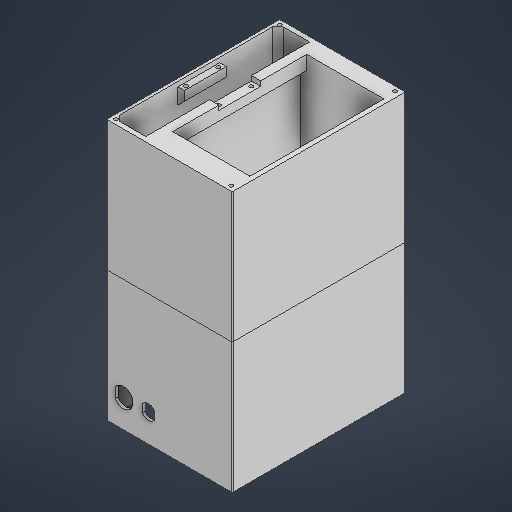
# Autodesk Inventor part: Kameraturm
Saved by Autodesk Inventor 2026.1 (Build 301233020, 233B)
## iProperties
Created: 2025-08-17
Part Number: Kameraturm
Material: Generic
Document SubType Name: Modeling
Designer: peter
Density: 1 g/cm^3
Appearance: Default
Author: peter
Autodesk Inventor part; units mm, degrees
ref_plane "YZ Plane" through (0, 0, 0) normal (1, 0, 0) x (0, 1, 0)
ref_plane "XZ Plane" through (0, 0, 0) normal (0, 1, 0) x (-1, 0, 0)
sketch "Sketch1" plane through (0, 0, 0) normal (0, 0, 1) x (1, 0, 0)
  line L0 (-67.5, -90) -> (67.5, -90)
  line L1 (67.5, -90) -> (67.5, 93)
  line L2 (67.5, 93) -> (-67.5, 93)
  line L3 (-67.5, 93) -> (-67.5, -90)
  line L4 (67.5, -90) -> (-67.5, -90)
  line L5 (-67.5, -90) -> (-67.5, -93)
  line L6 (-67.5, -93) -> (67.5, -93)
  line L7 (67.5, -93) -> (67.5, -90)
  line L8 (-67, -93) -> (-67.5, -92.5) projected
  line L9 (-67, -93) -> (67, -93) projected
  line L10 (67.5, -92.5) -> (67, -93) projected
  line L11 (67.5, -92.5) -> (67.5, 92.5) projected
  line L12 (67, 93) -> (67.5, 92.5) projected
  line L13 (67, 93) -> (-67, 93) projected
  line L14 (-67.5, 92.5) -> (-67, 93) projected
  line L15 (-67.5, 92.5) -> (-67.5, -92.5) projected
  circle A0 centre (57.5, 84) radius 7.05 projected
  circle A1 centre (57.5, -84) radius 7.05 projected
  circle A2 centre (-47.5, 0) radius 7.05 projected
  line L16 (62.5, 75) -> (62.5, -69) projected
  line L17 (62.5, -69) -> (-27.5, -69) projected
  line L18 (-27.5, -69) -> (-27.5, 75) projected
  line L19 (-27.5, 75) -> (62.5, 75) projected
  point P0 (0, 0)
  dimension "d17" = 3
  constraints: 16 end point, 4 parallel, 2 horizontal, 2 perpendicular, 1 coincident
  measures "d17" distance of L5.end L4.end
extrude "Extrusion1" add sketch "Sketch1" along normal blind 280 contours L3 L14 L2 L12 L1 L0 A1 | L0 A1 L7 L10 L6 L8 L5 | A1 L0 | L0 A1 | L3 L2 L14 | L8 L6 L5 | L2 L1 L12 | L10 L7 L6 | A0 | A2 | L16 L17 L18 L19
sketch "Sketch2" plane through (-67.5, -93, 0) normal (0, -1, 0) x (1, 0, 0)
  circle A0 centre (18, -18) radius 10.35 projected
  circle A1 centre (45, -18) radius 7.85 projected
  line L0 (18, -18) -> (18, 64.5706) construction
  line L1 (45, -18) -> (45, 64.5706) construction
  line L2 (40, 0) -> (40, 300) construction
  circle A2 centre (18, 30) radius 10.35
  circle A3 centre (45, 30) radius 7.85
  line L3 (0, 0) -> (135, 0) construction
  point P0 (67.5, 0)
  dimension "d2" = 30
  constraints: 4 end point, 2 centre point, 2 equal radius, 2 point on line, 1 horizontal alignment, 1 parallel, 1 vertical
  measures "d2" distance from line of L3 A2.centre
extrude "Extrusion3" cut sketch "Sketch2" against normal blind 8 contours A2 | A3
ref_plane "Work Plane2" through (0, 0, 34) normal (0, 0, -1) x (-1, 0, 0)
sketch "Sketch5" plane through (0, 0, 0) normal (0, 0, -1) x (-1, 0, 0)
  line L0 (27.5, 75) -> (-62.5, 75)
  line L1 (-62.5, 75) -> (-62.5, -69)
  line L2 (-62.5, -69) -> (27.5, -69)
  line L3 (27.5, -69) -> (27.5, 75)
  line L4 (-67.5, -92.5) -> (-67.5, 92.5)
  line L5 (-67.5, 92.5) -> (-67, 93)
  line L6 (-67, 93) -> (67, 93)
  line L7 (67, 93) -> (67.5, 92.5)
  line L8 (67.5, 92.5) -> (67.5, -92.5)
  line L9 (67.5, -92.5) -> (67, -93)
  line L10 (67, -93) -> (-67, -93)
  line L11 (-67, -93) -> (-67.5, -92.5)
  circle A0 centre (-57.5, 84) radius 7.05
  circle A1 centre (-57.5, -84) radius 7.05
  circle A2 centre (47.5, 0) radius 7.05
  point P0 (0, 0)
  constraints: 24 end point, 4 horizontal, 4 vertical, 3 centre point, 22 other
extrude "Extrusion5" cut sketch "Sketch5" against normal blind 300 contours L3 L2 L1 L0
sketch "Sketch6" plane through (0, 0, 0) normal (0, 0, -1) x (-1, 0, 0)
  line L0 (64.5, -90) -> (30.5, -90)
  line L1 (30.5, -90) -> (30.5, -55)
  line L2 (30.5, -55) -> (64.5, -55)
  line L3 (64.5, -55) -> (64.5, -90)
  line L4 (30.5, -90) -> (12.5, -90)
  line L5 (12.5, -90) -> (12.5, -72)
  line L6 (12.5, -72) -> (30.5, -72)
  line L7 (30.5, -72) -> (30.5, -90)
  line L8 (67.5, 93) -> (67.5, -93) projected
  line L9 (67.5, -93) -> (-67.5, -93) projected
  line L10 (27.5, -69) -> (-62.5, -69) projected
  line L11 (27.5, 75) -> (27.5, -69) projected
  point P0 (0, 0)
  dimension "d20" = 3
  dimension "d21" = 3
  dimension "d22" = 3
  dimension "d23" = 3
  dimension "d24" = 35
  dimension "d25" = 18
  constraints: 16 end point, 4 parallel, 2 horizontal, 2 perpendicular
  measures "d20" distance between parallel lines of L8 L3
  measures "d21" distance between parallel lines of L9 L0
  measures "d22" distance between parallel lines of L10 L6
  measures "d23" distance between parallel lines of L11 L1
  measures "d24" distance between parallel lines of L0 L2
  measures "d25" distance between parallel lines of L1 L5
extrude "Extrusion6" cut sketch "Sketch6" against normal blind 55
sketch "Sketch7" plane through (0, 0, 55) normal (0, 0, -1) x (-1, 0, 0)
  line L0 (64.5, -55) -> (64.5, -90) projected
  line L1 (64.5, -88) -> (30.5, -88)
  line L2 (30.5, -88) -> (30.5, 88)
  line L3 (30.5, 88) -> (64.5, 88)
  line L4 (64.5, 88) -> (64.5, -88)
  line L5 (67.5, -93) -> (-67.5, -93) projected
  line L6 (27.5, -69) -> (27.5, 75) projected
  line L7 (-67.5, 93) -> (67.5, 93) projected
  point P0 (0, 0)
  point P1 (47.5, -88)
  dimension "d28" = 5
  dimension "d29" = 3
  dimension "d30" = 5
  constraints: 8 end point, 2 parallel, 1 horizontal, 1 midpoint, 1 perpendicular, 1 point on line
  measures "d28" distance from line of L5 point (47.5, -88)
  measures "d29" distance between parallel lines of L6 L2
  measures "d30" distance between parallel lines of L7 L3
extrude "Extrusion7" cut sketch "Sketch7" against normal through all
chamfer "Chamfer2" distance 6 angle 45 2 edges at (-64.5, 88, 167.5) (-64.5, -88, 167.5)
sketch "Sketch8" plane through (0, 0, 280) normal (0, 0, 1) x (1, 0, 0)
  line L0 (-27.5, 75) -> (62.5, 75) projected
  line L1 (17.5, 75) -> (17.5, -69) construction
  line L2 (62.5, -69) -> (-27.5, -69) projected
  line L3 (-30.5, -90.6404) -> (-20.5, -90.6404)
  line L4 (-20.5, -90.6404) -> (-20.5, 89.3596)
  line L5 (-20.5, 89.3596) -> (-30.5, 89.3596)
  line L6 (-30.5, 89.3596) -> (-30.5, -90.6404)
  line L7 (-30.5, -90.6404) -> (-20.5, 89.3596) construction
  line L8 (-20.5, -90.6404) -> (-30.5, 89.3596) construction
  line L9 (-27.5, -69) -> (-27.5, 75) projected
  line L10 (-67.5, -19.5) -> (-57.5, -19.5)
  line L11 (-57.5, -19.5) -> (-57.5, 25.5)
  line L12 (-57.5, 25.5) -> (-67.5, 25.5)
  line L13 (-67.5, 25.5) -> (-67.5, -19.5)
  line L14 (-67.5, -19.5) -> (-57.5, 25.5) construction
  line L15 (-57.5, -19.5) -> (-67.5, 25.5) construction
  line L16 (-67.5, 93) -> (-67.5, -93) projected
  point P0 (0, 0)
  point P1 (17.5, 3)
  point P2 (-62.5, 3)
  point P3 (-30.5, 88)
  dimension "d36" = 10
  dimension "d37" = 180
  dimension "d39" = 10
  dimension "d40" = 45
  constraints: 26 end point, 5 midpoint, 4 parallel, 2 horizontal, 2 perpendicular, 2 point on line, 1 horizontal alignment
  measures "d36" distance of L5.end L4.end
  measures "d37" distance of L4.end L3.end
  measures "d39" distance of L12.end L11.end
  measures "d40" distance of L11.end L10.end
extrude "Extrusion8" add sketch "Sketch8" against normal blind 15
chamfer "Chamfer3" distance 7 angle 45 1 edges at (-64.5, 3, 265)
chamfer "Chamfer5" distance 7 angle 45 1 edges at (-27.5, 3, 265)
sketch "Sketch9" plane through (0, 0, 280) normal (0, 0, 1) x (1, 0, 0)
  line L0 (-64.5, -55) -> (-64.5, 82) projected
  line L1 (-64.5, 25.5) -> (-10.6333, 25.5)
  line L2 (-10.6333, 25.5) -> (-10.6333, -19.5)
  line L3 (-10.6333, -19.5) -> (-64.5, -19.5)
  line L4 (-64.5, -19.5) -> (-64.5, 25.5)
  line L5 (-57.5, -19.5) -> (-57.5, 25.5) projected
  point P0 (0, 0)
  point P1 (-10.6333, 3)
  point P2 (-57.5, 3)
  dimension "d52" = 45
  constraints: 8 end point, 2 midpoint, 2 parallel, 1 horizontal, 1 horizontal alignment, 1 perpendicular, 1 point on line
  measures "d52" distance of L1.end L2.end
extrude "Extrusion9" cut sketch "Sketch9" against normal blind 5
sketch "Sketch10" plane through (0, 0, 275) normal (0, 0, 1) x (1, 0, 0)
  line L0 (-57.5, 25.5) -> (-57.5, -19.5) projected
  line L1 (-57.5, 3) -> (-30.5, 3) construction
  line L2 (-30.5, -19.5) -> (-30.5, 25.5) projected
  line L3 (-64.5, 25.5) -> (-57.5, 25.5) projected
  line L4 (-61, 25.5) -> (-61, -19.5) construction
  line L5 (-30.5, 25.5) -> (-20.5, 25.5) projected
  line L6 (-25.5, 25.5) -> (-25.5, -19.5) construction
  line L7 (-20.5, -19.5) -> (-30.5, -19.5) projected
  point P0 (0, 0)
  point P1 (-61, 20.5)
  point P2 (-61, -14.5)
  point P3 (-25.5, 20.5)
  point P4 (-25.5, -14.5)
  dimension "d55" = 35
  constraints: 6 end point, 5 midpoint, 2 point on line, 2 symmetric about line, 1 horizontal alignment, 1 vertical
  measures "d55" distance of point (-25.5, -14.5) point (-25.5, 20.5)
hole "Hole1" at (-61, 20.5, 275) at (-61, -14.5, 275) at (-25.5, 20.5, 275) at (-25.5, -14.5, 275) direction (0, 0, -1) diameter 4 depth 8
sketch "Sketch11" plane through (0, 0, 280) normal (0, 0, 1) x (1, 0, 0)
  line L0 (67.5, 93) -> (-67.5, 93) projected
  line L1 (-67.5, 93) -> (-67.5, -93) projected
  point P0 (0, 0)
  point P1 (-62.5, 88)
  point P2 (-62.5, -87.8536)
  point P3 (61.2932, -87.8536)
  point P4 (61.2932, 88)
  dimension "d63" = 5
  dimension "d64" = 5
  constraints: 2 horizontal alignment, 2 vertical alignment
  measures "d63" distance from line of L0 point (-62.5, 88)
  measures "d64" distance from line of L1 point (-62.5, 88)
hole "Hole2" at (-62.5, 88, 280) at (-62.5, -87.8536, 280) at (61.2932, -87.8536, 280) at (61.2932, 88, 280) direction (0, 0, -1) diameter 4 depth 15
sketch "Skizze12" plane through (-67.5, -93, 0) normal (0, -1, 0) x (1, 0, 0)
  arc A0 (26.82, -17.5366) -> (26.82, -28.4634) centre (18, -23) ccw projected
  line L0 (26.82, -28.4634) -> (26.82, -17.5366) projected
  circle A1 centre (18, 30) radius 10.35 projected
  circle A2 centre (45, 30) radius 7.85 projected
  arc A3 (51.775, -18.6524) -> (38.225, -18.6524) centre (45, -23) ccw projected
  arc A4 (38.225, -27.3476) -> (41.0248, -30) centre (45, -23) ccw projected
  line L1 (38.225, -18.6524) -> (38.225, -27.3476) projected
  line L2 (41.0248, -30) -> (51.775, -18.6524)
  line L3 (9.2094, 35.4634) -> (9.2094, 24.5366)
  circle A5 centre (18, 30) radius 10.35 projected
  line L4 (38.4639, 34.3476) -> (38.4639, 25.6524)
  line L5 (130, 0) -> (40, 0) projected
  line L6 (45.7338, 37.8156) -> (45.7338, 22.1844)
  line L7 (135, 0) -> (0, 0) projected
  circle A6 centre (18, 50) radius 10.35
  circle A7 centre (45, 50) radius 7.85
  line L8 (9.2094, 55.4634) -> (9.2094, 44.5366)
  line L9 (38.4639, 54.3476) -> (38.4639, 45.6524)
  line L10 (51.5361, 54.3476) -> (51.5361, 45.6524)
  line L11 (51.5361, 34.3476) -> (51.5361, 25.6524)
  point P0 (67.5, 0)
  point P1 (15.3312, 40)
  point P2 (20.6688, 40)
  point P3 (15.3312, 40)
  point P4 (20.6688, 40)
  dimension "d98" = 20
  constraints: 16 end point, 14 point on circle, 4 vertical, 4 vertical alignment, 3 equal length, 3 horizontal alignment, 2 centre point, 2 equal radius, 2 perpendicular, 1 parallel
  measures "d98" distance of A1.centre A6.centre
extrude "Extrusion10" add sketch "Skizze12" against normal up to surface (3 mm away) contours L3 A1 | A2 L11 | L4 A2
sketch "Skizze13" plane through (-64.5, -90, 0) normal (1, 0, 0) x (0, 0, -1)
  line L0 (-280, 8) -> (-280, 172) projected
  line L1 (-55, 8) -> (-280, 8) projected
  line L2 (-55, 8) -> (-55, 0) projected
  line L3 (0, 0) -> (-55, 0) projected
  line L4 (0, 35) -> (0, 0) projected
  line L5 (0, 35) -> (-55, 35) projected
  line L6 (-55, 35) -> (-55, 172) projected
  line L7 (-280, 172) -> (-55, 172) projected
  line L8 (-275, 70.5) -> (-275, 115.5) projected
  line L9 (-275, 115.5) -> (-258, 115.5) projected
  line L10 (-258, 70.5) -> (-258, 115.5) projected
  line L11 (-258, 70.5) -> (-275, 70.5) projected
  line L12 (-2, 7.5) -> (-4, 7.5)
  line L13 (-4, 7.5) -> (-4, 27.5)
  line L14 (-4, 27.5) -> (-2, 27.5)
  line L15 (-2, 27.5) -> (-2, 7.5)
  point P0 (0, 90)
  point P1 (-2, 17.5)
  point P2 (-4, 17.5)
  point P3 (0, 17.5)
  dimension "d74" = 2
  dimension "d75" = 20
  dimension "d76" = 2
  constraints: 8 end point, 3 midpoint, 2 parallel, 1 horizontal, 1 horizontal alignment, 1 perpendicular
  measures "d74" distance of L13.end L14.end
  measures "d75" distance of L12.end L13.end
  measures "d76" distance from line of L4 point (-2, 17.5)
extrude "Extrusion11" cut sketch "Skizze13" against normal blind 2 contours L12 L13 L14 L15
sketch "Skizze14" plane through (0, 0, 0) normal (0, 0, -1) x (-1, 0, 0)
  line L0 (22.5, -86) -> (2.5, -86)
  line L1 (2.5, -86) -> (2.5, -76)
  line L2 (2.5, -76) -> (22.5, -76)
  line L3 (22.5, -76) -> (22.5, -86)
  line L4 (12.5, -90) -> (12.5, -72) projected
  line L5 (22.5, -86) -> (2.5, -76) construction
  line L6 (2.5, -86) -> (22.5, -76) construction
  point P0 (0, 0)
  point P1 (12.5, -81)
  point P2 (12.5, -86)
  point P3 (12.5, -76)
  dimension "d79" = 20
  dimension "d80" = 10
  constraints: 12 end point, 3 midpoint, 2 parallel, 1 horizontal, 1 perpendicular
  measures "d79" distance of L1.end L2.end
  measures "d80" distance of L0.end L1.end
extrude "Extrusion12" cut sketch "Skizze14" against normal blind 4 contours L0 L1 L2 L4
sketch "Skizze15" plane through (0, 0, 4) normal (0, 0, -1) x (-1, 0, 0)
  line L0 (2.5, -86) -> (2.5, -76) projected
  line L1 (12.5, -86) -> (2.5, -86) projected
  point P0 (0, 0)
  point P1 (7.5, -81)
  point P2 (2.5, -81)
  point P3 (7.5, -86)
  constraints: 2 midpoint, 1 horizontal alignment, 1 vertical alignment
hole "Bohrung3" at (-7.5, -81, 4) direction (0, 0, 1) diameter 4 depth 8
chamfer "Fasen6" distance 1 angle 45 4 edges at (67.5, -93, 140) (67.5, 93, 140) (-67.5, 93, 140) (-67.5, -93, 140)
sketch "Skizze16" plane through (0, 0, 0) normal (0, 0, -1) x (-1, 0, 0)
  circle A0 centre (47.5, 0) radius 7.05 projected
  circle A1 centre (-57.5, -84) radius 7.05 projected
  circle A2 centre (-57.5, 84) radius 7.05 projected
  point P0 (0, 0)
extrude "Extrusion13" cut sketch "Skizze16" against normal blind 4.5
ref_plane "Arbeitsebene3" through (0, 0, 140) normal (0, 0, 1) x (1, 0, 0)
split body "Trennen1" result two bodies by plane through (0, 0, 140) normal (0, 0, 1) first body at (-67, -30.6667, 233.3333)
chamfer "Fasen7" distance 0.5 angle 45 3 edges at (64.55, -84, 0) (-40.45, 0, 0) (64.55, 84, 0)
sketch "Skizze17" plane through (-66.5, -93, 140) normal (0, 0, 1) x (1, 0, 0)
  circle A0 centre (72.0741, 176.8933) radius 2
  circle A1 centre (97.6405, 11.2247) radius 2
  point P0 (66.5, 93)
  dimension "d99" = 4
  dimension "d100" = 4
  constraints: 2 centre point
  measures "d99" diameter of A0
  measures "d100" diameter of A1
extrude "Extrusion14" cut sketch "Skizze17" along normal mid plane 15 bodies 3 2
